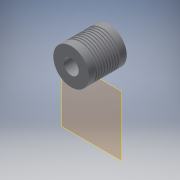
# Autodesk Inventor part: smaller
Saved by Autodesk Inventor 2019 (Build 230136000, 136)
## iProperties
Created: 2021-03-26
Part Number: smaller
Material: Generic
Document SubType Name: Modeling
Designer: Ian
Density: 1 g/cm^3
Appearance: Default
Author: Ian
Autodesk Inventor part; units mm, degrees
ref_plane "YZ Plane" through (0, 0, 0) normal (1, 0, 0) x (0, 1, 0)
ref_plane "XZ Plane" through (0, 0, 0) normal (0, 1, 0) x (-1, 0, 0)
ref_plane "XY Plane" through (0, 0, 0) normal (0, 0, 1) x (1, 0, 0)
ref_plane "Work Plane1" through (0, 0, 6.1) normal (0, 0, 1) x (1, 0, 0)
sketch "Sketch1" plane through (0, 0, 6.1) normal (0, 0, 1) x (1, 0, 0)
  circle A0 centre (0, 13.698) radius 2 construction
  circle A1 centre (0, 13.698) radius 2.2
  circle A2 centre (0, 13.698) radius 5.2
  point P0 (0, 0)
  dimension "d0" = 4
  dimension "d1" = 0.2
  dimension "d2" = 3
  constraints: 3 centre point, 1 vertical alignment
  measures "d0" diameter of A0
  measures "d1" radial gap between concentric circles of A0 A1
  measures "d2" radial gap between concentric circles of A1 A2
extrude "Extrusion1" add sketch "Sketch1" along normal blind 6 and the other way blind 5
sketch "Sketch3" plane through (0, 0, 0) normal (1, 0, 0) x (0, 1, 0)
  line L0 (8, 9.65) -> (8, 9.85) construction
  line L1 (8, 3.25) -> (8, 3.45) construction
  line L2 (8, 9.75) -> (18.898, 9.75) construction
  line L3 (18.898, 1.1) -> (18.898, 12.1) construction
  arc A0 (18.798, 10.05) -> (18.798, 9.45) centre (18.798, 9.75) ccw
  line L4 (18.798, 10.05) -> (18.898, 10.05)
  line L5 (18.898, 10.05) -> (18.898, 9.45)
  line L6 (18.898, 9.45) -> (18.798, 9.45)
  arc A1 (18.798, 9.25) -> (18.798, 8.65) centre (18.798, 8.95) ccw
  line L7 (18.898, 8.65) -> (18.798, 8.65)
  line L8 (18.898, 9.25) -> (18.898, 8.65)
  line L9 (18.798, 9.25) -> (18.898, 9.25)
  arc A2 (18.798, 8.45) -> (18.798, 7.85) centre (18.798, 8.15) ccw
  line L10 (18.898, 7.85) -> (18.798, 7.85)
  line L11 (18.898, 8.45) -> (18.898, 7.85)
  line L12 (18.798, 8.45) -> (18.898, 8.45)
  arc A3 (18.798, 7.65) -> (18.798, 7.05) centre (18.798, 7.35) ccw
  line L13 (18.898, 7.05) -> (18.798, 7.05)
  line L14 (18.898, 7.65) -> (18.898, 7.05)
  line L15 (18.798, 7.65) -> (18.898, 7.65)
  arc A4 (18.798, 6.85) -> (18.798, 6.25) centre (18.798, 6.55) ccw
  line L16 (18.898, 6.25) -> (18.798, 6.25)
  line L17 (18.898, 6.85) -> (18.898, 6.25)
  line L18 (18.798, 6.85) -> (18.898, 6.85)
  arc A5 (18.798, 6.05) -> (18.798, 5.45) centre (18.798, 5.75) ccw
  line L19 (18.898, 5.45) -> (18.798, 5.45)
  line L20 (18.898, 6.05) -> (18.898, 5.45)
  line L21 (18.798, 6.05) -> (18.898, 6.05)
  arc A6 (18.798, 5.25) -> (18.798, 4.65) centre (18.798, 4.95) ccw
  line L22 (18.898, 4.65) -> (18.798, 4.65)
  line L23 (18.898, 5.25) -> (18.898, 4.65)
  line L24 (18.798, 5.25) -> (18.898, 5.25)
  arc A7 (18.798, 4.45) -> (18.798, 3.85) centre (18.798, 4.15) ccw
  line L25 (18.898, 3.85) -> (18.798, 3.85)
  line L26 (18.898, 4.45) -> (18.898, 3.85)
  line L27 (18.798, 4.45) -> (18.898, 4.45)
  arc A8 (18.798, 3.65) -> (18.798, 3.05) centre (18.798, 3.35) ccw
  line L28 (18.898, 3.05) -> (18.798, 3.05)
  line L29 (18.898, 3.65) -> (18.898, 3.05)
  line L30 (18.798, 3.65) -> (18.898, 3.65)
  line L31 (8, 3.35) -> (18.898, 3.35) construction
  line L32 (18.898, 12.1) -> (8.498, 12.1) projected
  line L33 (13.698, 12.1) -> (13.698, 1.1)
  point P0 (0, 0)
  dimension "d18" = 0.6
  dimension "d19" = 0.1
  dimension "d22" = 0.8
  constraints: 64 end point, 18 point on circle, 9 centre point, 4 midpoint, 4 vertical, 3 perpendicular, 2 point on line, 2 tangent, 1 collinear, 1 horizontal, 76 other
  measures "d18" diameter of A0
  measures "d19" distance of L4.start L4.end
  measures "d22" distance of A0.centre A1.centre
revolve "Revolution2" cut sketch "Sketch3" angle 360 about axis through (0, 13.698, 12.1) along (0, 0, -1)
sketch "Sketch2" plane through (0, 0, 0) normal (1, 0, 0) x (0, 1, 0)
  line L0 (8.498, 1.1) -> (18.898, 1.1) projected
  line L1 (18.898, 12.1) -> (8.498, 12.1) projected
  line L2 (18.898, 1.1) -> (18.898, 12.1) projected
  line L3 (18.898, 9.975) -> (17.898, 9.225)
  line L4 (17.898, 9.225) -> (17.898, 8.975)
  line L5 (17.898, 8.975) -> (18.898, 8.225)
  line L6 (18.898, 8.225) -> (18.898, 7.975)
  line L7 (18.898, 7.975) -> (17.898, 7.225)
  line L8 (17.898, 7.225) -> (17.898, 6.975)
  line L9 (17.898, 6.975) -> (18.898, 6.225)
  line L10 (18.898, 6.225) -> (18.898, 5.975)
  line L11 (18.898, 5.975) -> (17.898, 5.225)
  line L12 (17.898, 5.225) -> (17.898, 4.975)
  line L13 (17.898, 4.975) -> (18.898, 4.225)
  line L14 (18.898, 4.225) -> (18.898, 3.975)
  line L15 (18.898, 3.975) -> (17.898, 3.225)
  line L16 (17.898, 3.225) -> (17.898, 2.975)
  line L17 (17.898, 2.975) -> (18.898, 2.225)
  line L18 (8, 2.975) -> (8, 3.225) construction
  line L19 (8, 3.225) -> (7, 3.975) construction
  line L20 (7, 2.225) -> (8, 2.975) construction
  line L21 (8, 2.975) -> (17.898, 2.975) construction
  line L22 (8, 2.975) -> (17.898, 2.975) construction
  line L23 (8, 3.225) -> (16.4909, 3.225) construction
  line L24 (18.898, 9.975) -> (18.898, 8.225) construction
  line L25 (18.898, 7.975) -> (18.898, 6.225)
  line L26 (18.898, 5.975) -> (18.898, 4.225) construction
  line L27 (18.898, 3.975) -> (18.898, 2.225)
  line L28 (18.898, 12.1) -> (8.498, 12.1) construction
  line L29 (8.498, 1.1) -> (18.898, 1.1) construction
  line L30 (18.898, 5.975) -> (18.898, 4.225)
  line L31 (18.898, 2.2341) -> (18.898, 9.975)
  line L32 (18.898, 1.1) -> (8.498, 1.1) construction
  line L33 (13.698, 1.1) -> (13.698, 9.975) construction
  point P0 (0, 0)
  dimension "d7" = 0.25
  dimension "d8" = 0.25
  dimension "d9" = 0.25
  dimension "d10" = 0.25
  dimension "d11" = 0.25
  dimension "d12" = 0.25
  dimension "d13" = 0.25
  dimension "d14" = 1
  dimension "d15" = 2
  dimension "d16" = 0
  constraints: 58 end point, 12 point on line, 8 parallel, 6 collinear, 2 equal length, 2 horizontal, 2 vertical, 1 midpoint, 1 perpendicular, 6 other
  measures "d7" distance of L3.end L4.end
  measures "d8" distance of L5.end L6.end
  measures "d9" distance of L7.end L8.end
  measures "d10" distance of L9.end L10.end
  measures "d11" distance of L11.end L12.end
  measures "d12" distance of L13.end L14.end
  measures "d13" distance of L15.end L16.end
  measures "d14" distance between parallel lines of L2 L4
  measures "d15" distance of L6.end L3.start
  measures "d16" distance between parallel lines of L21 L22
body "Solid1"
